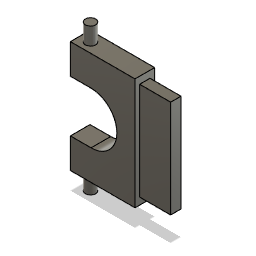
Tuf_K3_keyboard_spacer (Autodesk Fusion 360 design; units mm, degrees)
Autodesk Fusion 360 part; units mm, degrees
sketch "Sketch1" plane through (0, 0, 0) normal (0, 1, 0) x (1, 0, 0)
  line L0 (0, 0) -> (-12.5, 0)
  line L1 (-12.5, 0) -> (-12.5, 3.8)
  line L2 (-12.5, 3.8) -> (0, 3.8)
  line L3 (0, 3.8) -> (0, 2.9)
  line L4 (0, 2.9) -> (6, 2.9)
  line L5 (6, 2.9) -> (6, 0.9)
  line L6 (6, 0.9) -> (0, 0.9)
  line L7 (0, 0) -> (0, 0.9)
  line L8 (6, 0.9) -> (6, 2.9)
  line L9 (6, 2.9) -> (0, 2.9)
  line L10 (0, 3.8) -> (-12.5, 3.8)
  circle A0 centre (-10.5, 1.9) radius 1
  line L11 (0, 2.9) -> (0, 0.9)
  dimension "d1" = 12.5
  dimension "d2" = 3.8
  dimension "d4" = 6
  dimension "d5" = 2
  dimension "d8" = 2
  constraint horizontal L0
  constraint vertical L1
  constraint horizontal L2
  constraint coincident L0.start L7.start
  constraint perpendicular L2 L3
  constraint horizontal L4
  constraint vertical L5
  constraint horizontal L6
  constraint perpendicular L6 L7
  constraint perpendicular L6 L11
  measures "d1" distance of L0.start L0.end
  measures "d2" distance of L0.start L2.end
  measures "d4" distance of L3.end L4.end
  measures "d5" distance of L4.end L5.end
  measures "d8" diameter of A0
extrude "Extrude1" add sketch "Sketch1" along normal blind 10.8 contours L0 L1 L2 L3 L7 L10 L11 makes body 1
extrude "Extrude2" add sketch "Sketch1" along normal blind 9.45 contours L4 L5 L6 L8 L9 L11 bodies 1
extrude "Extrude3" add sketch "Sketch1" along normal blind 14.15 separate body contours A0 makes body 2
sketch "Sketch2" plane through (0, 0, 0) normal (0, 0, 1) x (1, 0, 0)
  line L0 (-12.5, 0) -> (0, 0)
  line L1 (0, 0) -> (0, 10.8)
  line L2 (0, 10.8) -> (-12.5, 10.8)
  line L3 (-12.5, 10.8) -> (-12.5, 0)
  line L4 (-12.5, 10.8) -> (-12.5, 5)
  arc A0 (-3.5, 0) -> (-8.5, 5) centre (-8.5, 0) ccw
  line L5 (-8.5, 5) -> (-12.5, 5)
  line L6 (-3.5, 0) -> (-12.5, 0)
  line L7 (-12.5, 0) -> (-12.5, 5)
  dimension "d15" = 5.8
  constraint coincident L2.end L3.start
  constraint perpendicular L2 L4
  constraint coincident L0 A0.start
  constraint tangent A0 L5
  constraint coincident L0.start L3.end
  constraint perpendicular L5 L7
  measures "d15" distance of L2.end L4.end
extrude "Extrude4" cut sketch "Sketch2" against normal blind 9 contours L0 L3 A0 L5 L6 L7 bodies 1 2
combine "Combine1" operation add target body 1 tool bodies 2
mirror "Mirror1" about plane through (0, 0, 0) normal (0, -1, 0) of bodies 1 merged
